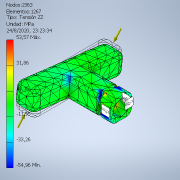
# Autodesk Inventor part: T_CORREGIDA
Saved by Autodesk Inventor 2020.3 (Build 243373000, 373)
## iProperties
Created: 2020-01-10
Part Number: T_CORREGIDA
Material: Resina termoplástica
Document SubType Name: Modeling
Designer: Laptop
Density: 1.28 g/cm^3
Appearance: Suave - Negro
Author: Laptop
Autodesk Inventor part; units mm, degrees
ref_plane "YZ Plane" through (0, 0, 0) normal (1, 0, 0) x (0, 1, 0)
ref_plane "XZ Plane" through (0, 0, 0) normal (0, 1, 0) x (-1, 0, 0)
ref_plane "XY Plane" through (0, 0, 0) normal (0, 0, 1) x (1, 0, 0)
sketch "Boceto1" plane through (0, 0, 0) normal (0, 0, 1) x (1, 0, 0)
  line L0 (0, 0) -> (20, 0)
  line L1 (20, 0) -> (20, -20)
  line L2 (20, -20) -> (0, -20)
  line L3 (0, -20) -> (0, 0)
  dimension "d0" = 20
  dimension "d1" = 20
  constraints: 8 end point, 2 parallel, 1 horizontal, 1 perpendicular
  measures "d0" distance of L1.end L2.end
  measures "d1" distance of L0.end L1.end
extrude "Extrusión1" add sketch "Boceto1" along normal blind 90
fillet "Empalme1" radius 5 4 edges at (0, 0, 45) (20, 0, 45) (20, -20, 45) (0, -20, 45)
fillet "Empalme2" radius 7 16 edges at (1.4645, -1.4645, 90) (0, -10, 90) (1.4645, -18.5355, 90) (10, -20, 90) (18.5355, -18.5355, 90) (20, -10, 90) (18.5355, -1.4645, 90) (10, 0, 90) (10, 0, 0) (1.4645, -1.4645, 0) (0, -10, 0) (1.4645, -18.5355, 0) (10, -20, 0) (18.5355, -18.5355, 0) (20, -10, 0) (18.5355, -1.4645, 0)
ref_plane "Plano de trabajo1" through (10, -15, 7) normal (1, 0, 0) x (0, 0, -1)
sketch "Boceto2" plane through (10, -15, 7) normal (1, 0, 0) x (0, 0, -1)
  line L0 (-76, 15) -> (0, 15) projected
  line L1 (-38, 15) -> (-38, 5)
  line L2 (-48, 15) -> (-28, 15)
  line L3 (-28, 15) -> (-28, -5)
  line L4 (-28, -5) -> (-48, -5)
  line L5 (-48, -5) -> (-48, 15)
  line L6 (-48, 15) -> (-28, -5) construction
  line L7 (-28, 15) -> (-48, -5) construction
  point P0 (7, 15)
  dimension "d7" = 10
  dimension "d8" = 20
  dimension "d9" = 20
  constraints: 14 end point, 3 midpoint, 2 parallel, 1 horizontal, 1 perpendicular, 1 vertical
  measures "d7" distance of L1.start L1.end
  measures "d8" distance of L3.end L4.end
  measures "d9" distance of L2.end L3.end
extrude "Extrusión2" add sketch "Boceto2" along normal blind 50
fillet "Empalme3" radius 5 4 edges at (37.5, 0, 35) (37.5, 0, 55) (37.5, -20, 55) (37.5, -20, 35)
ref_plane "Plano de trabajo2" through (50, -15, 7) normal (1, 0, 0) x (0, 0, -1)
sketch "Boceto3" plane through (60, -15, 7) normal (1, 0, 0) x (0, 0, -1)
  line L0 (-43, -5) -> (-33, -5) projected
  line L1 (-38, -5) -> (-38, 5)
  circle A0 centre (-38, 5) radius 7.6
  point P0 (7, 15)
  dimension "d14" = 10
  dimension "d15" = 15.2
  constraints: 2 end point, 1 centre point, 1 coincident, 1 midpoint, 1 vertical
  measures "d14" distance of L1.start L1.end
  measures "d15" diameter of A0
extrude "Extrusión3" cut sketch "Boceto3" against normal blind 30
sketch "Boceto4" plane through (50, -15, 7) normal (1, 0, 0) x (0, 0, -1)
  line L0 (-38, 5) -> (-43, 5)
  line L1 (-38, 5) -> (-33, 5)
  arc A0 (-33, -7.9185) -> (-33, 17.9185) centre (-38, 5) ccw
  arc A1 (-43, 17.9185) -> (-43, -7.9185) centre (-38, 5) ccw
  circle A2 centre (-38, 5) radius 7.6 projected
  circle A3 centre (-38, 5) radius 7.6
  line L2 (-33, 17.9185) -> (-33, 10.7236)
  line L3 (-33, -7.9185) -> (-33, -0.7236)
  line L4 (-43, -7.9185) -> (-43, -0.7236)
  line L5 (-43, 17.9185) -> (-43, 10.7236)
  point P0 (7, 15)
  dimension "d28" = 5
  dimension "d29" = 5
  constraints: 12 end point, 8 point on circle, 3 centre point, 2 coincident, 2 horizontal, 2 point on line, 1 concentric, 1 parallel, 1 vertical
  measures "d28" distance of L0.start L0.end
  measures "d29" distance of L0.start L1.end
extrude "Extrusión4" cut sketch "Boceto4" against normal blind 3.8 contours L3 A2 L2 A0 | L4 A1 L5 A2
ref_plane "Plano de trabajo3" through (5, -10, 83) normal (0, -1, 0) x (1, 0, 0)
